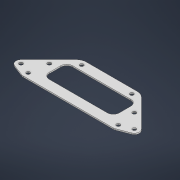
# Autodesk Inventor part: gusset-2-3.25-full
Saved by Autodesk Inventor 2021 (Build 250183000, 183)
## iProperties
Created: 2020-11-04
Part Number: gusset-2-3.25-full
Material: Generic
Document SubType Name: Modeling
Designer: Carlos Stewart
Density: 1 g/cm^3
Appearance: Default
Author: Carlos Stewart
Autodesk Inventor part; units mm, degrees
ref_plane "YZ Plane" through (0, 0, 0) normal (1, 0, 0) x (0, 1, 0)
ref_plane "XZ Plane" through (0, 0, 0) normal (0, 1, 0) x (-1, 0, 0)
ref_plane "XY Plane" through (0, 0, 0) normal (0, 0, 1) x (1, 0, 0)
sketch "Sketch1" plane through (0, 0, 0) normal (0, 1, 0) x (-1, 0, 0)
  line L0 (-37.8542, -1.1176) -> (35.8058, -1.1176)
  line L1 (43.4258, -8.7376) -> (43.4258, -23.2918)
  line L2 (35.8058, -30.9118) -> (-37.8542, -30.9118)
  line L3 (-45.4742, -23.2918) -> (-45.4742, -8.7376)
  arc A0 (-37.8542, -1.1176) -> (-45.4742, -8.7376) centre (-37.8542, -8.7376) ccw
  arc A1 (-45.4742, -23.2918) -> (-37.8542, -30.9118) centre (-37.8542, -23.2918) ccw
  arc A2 (35.8058, -30.9118) -> (43.4258, -23.2918) centre (35.8058, -23.2918) ccw
  arc A3 (43.4258, -8.7376) -> (35.8058, -1.1176) centre (35.8058, -8.7376) ccw
  circle A4 centre (-72.8662, -0.3634) radius 2.3114
  circle A5 centre (-54.9057, -18.324) radius 2.3114
  circle A6 centre (-58.1742, 5.2324) radius 2.3114
  circle A7 centre (56.1258, 5.2324) radius 2.3114
  circle A8 centre (-32.7742, -37.2618) radius 2.3114
  circle A9 centre (30.7258, -37.2618) radius 2.3114
  circle A10 centre (52.8574, -18.324) radius 2.3114
  circle A11 centre (70.8179, -0.3634) radius 2.3114
  arc A12 (75.308, -4.8536) -> (73.078, 5.5707) centre (70.8179, -0.3634) ccw
  arc A13 (58.386, 11.1665) -> (56.1258, 11.5824) centre (56.1258, 5.2324) ccw
  arc A14 (30.7258, -43.6118) -> (30.9592, -43.6075) centre (30.7258, -37.2618) ccw
  arc A15 (-75.1264, 5.5707) -> (-77.3564, -4.8536) centre (-72.8662, -0.3634) ccw
  arc A16 (-59.3959, -22.8141) -> (-59.0342, -23.1487) centre (-54.9057, -18.324) ccw
  arc A17 (-33.0076, -43.6075) -> (-32.7742, -43.6118) centre (-32.7742, -37.2618) ccw
  arc A18 (-58.1742, 11.5824) -> (-60.4344, 11.1665) centre (-58.1742, 5.2324) ccw
  line L4 (-60.4344, 11.1665) -> (-75.1264, 5.5707)
  line L5 (-77.3564, -4.8536) -> (-42.3179, -39.8921)
  line L6 (-59.2215, -22.9884) -> (-59.0342, -23.1487)
  line L7 (58.386, 11.1665) -> (73.078, 5.5707)
  line L8 (75.308, -4.8536) -> (40.2695, -39.8921)
  line L9 (56.1258, 11.5824) -> (-58.1742, 11.5824)
  line L10 (31.2893, -43.6118) -> (-33.3376, -43.6118)
  arc A19 (31.2893, -43.6118) -> (40.2695, -39.8921) centre (31.2893, -30.9118) ccw
  arc A20 (-42.3179, -39.8921) -> (-33.3376, -43.6118) centre (-33.3376, -30.9118) ccw
  line L11 (35.8058, -30.9118) -> (-37.8542, -30.9118)
  point P0 (0, 0)
  point P1 (43.4258, -30.9118)
  point P2 (-45.4742, -30.9118)
  point P3 (43.4258, -30.9118)
  dimension "d2" = 7.62
  dimension "d20" = 12.7
  dimension "d21" = 12.7
  dimension "d24" = 29.7942
  constraints: 28 point on circle, 26 tangent, 24 end point, 21 centre point, 8 coincident, 8 point on line, 3 equal length, 3 equal radius, 2 horizontal, 1 perpendicular, 15 other
  measures "d2" radius of A0
  measures "d20" radius of A19
  measures "d21" radius of A20
  measures "d24" distance between parallel lines of L2 L0
extrude "Extrusion1" add sketch "Sketch1" along normal blind 1.5875 contours L8 A19 L10 A20 L5 L6 A16 A15 L4 A18 L9 A13 L7 A12
body "Solid1"
